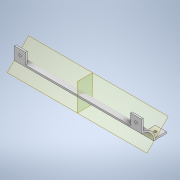
# Autodesk Inventor part: CableCoverForFrameHigher
Saved by Autodesk Inventor 2021 (Build 250183000, 183)
## iProperties
Created: 2021-05-28
Part Number: CableCoverForFrameHigher
Material: 一般
Document SubType Name: Modeling
Designer: gisen
Density: 1 g/cm^3
Appearance: 既定
Author: gisen
Autodesk Inventor part; units mm, degrees
ref_plane "YZ Plane" through (0, 0, 0) normal (1, 0, 0) x (0, 1, 0)
ref_plane "XZ Plane" through (0, 0, 0) normal (0, 1, 0) x (-1, 0, 0)
ref_plane "XY Plane" through (0, 0, 0) normal (0, 0, 1) x (1, 0, 0)
sketch "スケッチ1" plane through (0, 0, 0) normal (0, 1, 0) x (-1, 0, 0)
  line L0 (0, -22) -> (230, -22)
  line L1 (230, -22) -> (230, -25)
  line L2 (230, -25) -> (0, -25)
  line L3 (0, -25) -> (0, -22)
  line L4 (276, 0) -> (-46, 0) projected
  point P0 (0, 0)
  dimension "d0" = 3
  dimension "d1" = 230
  dimension "d2" = 25
  constraints: 8 end point, 2 parallel, 1 horizontal, 1 perpendicular
  measures "d0" distance of L2.end L0.start
  measures "d1" distance of L1.end L2.end
  measures "d2" distance of point (0, 0) L2.end
revolve "回転1" add sketch "スケッチ1" angle 90 about axis through (-10, 0, 0) along (1, 0, 0)
sketch "スケッチ2" plane through (-230, 25, 0) normal (0, 0, 1) x (1, 0, 0)
  line L0 (230, 0) -> (0, 0) projected
  line L1 (0, 0) -> (0, -3) projected
  line L2 (0, -3) -> (230, -3) projected
  line L3 (230, -3) -> (230, 0) projected
  line L4 (230, 0) -> (0, 0) projected
  line L5 (0, 0) -> (20, 0)
  line L6 (20, 0) -> (20, 20)
  line L7 (20, 20) -> (0, 20)
  line L8 (0, 20) -> (0, 0)
  line L9 (115, 0) -> (115, -3)
  line L10 (0, -3) -> (230, -3) projected
  line L11 (20, 0) -> (20, -3)
  circle A0 centre (10, 10) radius 2.25
  point P0 (230, -25)
  point P1 (20, 0)
  point P2 (20, -3)
  point P3 (20, 0)
  dimension "d4" = 20
  dimension "d5" = 20
  dimension "d8" = 4.5
  constraints: 12 end point, 2 midpoint, 2 parallel, 2 perpendicular, 1 centre point, 1 horizontal, 1 point on line
  measures "d4" distance of L7.end L0.end
  measures "d5" distance of L6.end L7.end
  measures "d8" diameter of A0
extrude "押し出し1" add sketch "スケッチ2" against normal blind 3 contours L11 L2 L1 L0 | L0 L8 L7 L6
ref_plane "作業平面1" through (-115, 0, -25) normal (-1, 0, 0) x (0, 0, 1)
mirror "ミラー1" about plane through (-115, 0, -25) normal (-1, 0, 0) of "押し出し1"
ref_plane "作業平面2" through (-230, 0, 0) normal (0, 0.7071068, 0.7071068) x (-1, 0, 0)
mirror "ミラー2" about plane through (-230, 0, 0) normal (0, 0.7071068, 0.7071068) of "ミラー1"
